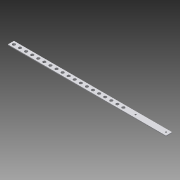
# Autodesk Inventor part: bottom clamper arm
Saved by Autodesk Inventor 2015 (Build 190159000, 159)
## iProperties
Created: 2015-03-29
Part Number: bottom clamper arm
Material: Aluminum 6061
Document SubType Name: Modeling
Designer: Jarod
Density: 2.7 g/cm^3
Appearance: Aluminum - Flat
Author: Jarod
Autodesk Inventor part; units mm, degrees
ref_plane "YZ Plane" through (0, 0, 0) normal (1, 0, 0) x (0, 1, 0)
ref_plane "XZ Plane" through (0, 0, 0) normal (0, 1, 0) x (-1, 0, 0)
ref_plane "XY Plane" through (0, 0, 0) normal (0, 0, 1) x (1, 0, 0)
sketch "Sketch1" plane through (0, 0, 0) normal (1, 0, 0) x (0, 1, 0)
  line L0 (0, 0) -> (-3.175, 0)
  line L1 (-3.175, 0) -> (-3.175, 25.4)
  line L2 (-3.175, 25.4) -> (0, 25.4)
  line L3 (0, 25.4) -> (0, 0)
  line L4 (0, 0) -> (-25.4, 0)
  line L5 (-25.4, 0) -> (-25.4, 3.175)
  line L6 (-25.4, 3.175) -> (0, 3.175)
  line L7 (0, 3.175) -> (0, 0)
  dimension "d0" = 3.175
  dimension "d1" = 25.4
  dimension "d2" = 25.4
  dimension "d3" = 3.175
  constraints: 16 end point, 4 parallel, 2 horizontal, 2 perpendicular
  measures "d0" distance of L1.end L2.end
  measures "d1" distance of L0.end L1.end
  measures "d2" distance of L5.end L6.end
  measures "d3" distance of L4.end L5.end
extrude "Extrusion1" add sketch "Sketch1" along normal blind 660.4
sketch "Sketch2" plane through (0, -25.4, 3.175) normal (0, 0, 1) x (1, 0, 0)
  line L0 (660.4, 22.225) -> (0, 22.225) projected
  line L1 (0, 22.225) -> (0, 0) projected
  line L2 (0, 0) -> (660.4, 0) projected
  line L3 (660.4, 22.225) -> (660.4, 0) projected
  line L4 (660.4, 0) -> (482.6, 0)
  line L5 (482.6, 0) -> (482.6, 22.225)
  line L6 (482.6, 22.225) -> (660.4, 22.225)
  line L7 (660.4, 22.225) -> (660.4, 0)
  point P0 (0, 25.4)
  dimension "d6" = 177.8
  dimension "d7" = 22.225
  constraints: 8 end point, 2 parallel, 1 horizontal, 1 perpendicular
  measures "d6" distance of L5.end L6.end
  measures "d7" distance of L4.end L5.end
extrude "Extrusion2" cut sketch "Sketch2" against normal blind 25.4 contours L3 L2 L5 L0
sketch "Sketch3" plane through (0, 0, 25.4) normal (0, 1, 0) x (1, 0, 0)
  line L0 (0, 25.4) -> (0, 0) projected
  line L1 (0, 0) -> (660.4, 0) projected
  line L2 (660.4, 25.4) -> (660.4, 0) projected
  line L3 (0, 25.4) -> (660.4, 25.4) projected
  point P0 (647.7, 12.7)
  point P1 (520.7, 12.7)
  dimension "d10" = 12.7
  dimension "d11" = 12.7
  dimension "d12" = 139.7
  dimension "d13" = 12.7
  measures "d10" distance from line of L3 point (647.7, 12.7)
  measures "d11" distance from line of L2 point (647.7, 12.7)
  measures "d12" distance from line of point (520.7, 12.7) L2
  measures "d13" distance from line of L3 point (520.7, 12.7)
hole "Hole1" at (647.7, 0, 12.7) at (520.7, 0, 12.7) direction (0, -1, 0) diameter 6.7469 end through all
sketch "Sketch4" plane through (0, -25.4, 0) normal (0, 0, -1) x (-1, 0, 0)
  line L0 (-660.4, 22.225) -> (-482.6, 22.225) projected
  line L1 (-482.6, 22.225) -> (-482.6, 0) projected
  line L2 (0, 0) -> (-482.6, 0) projected
  line L3 (0, 0) -> (0, 25.4) projected
  line L4 (0, 25.4) -> (-660.4, 25.4) projected
  line L5 (-660.4, 22.225) -> (-660.4, 25.4) projected
  line L6 (0, 0) -> (-482.6, 0)
  line L7 (-482.6, 0) -> (-482.6, 12.7)
  line L8 (-482.6, 12.7) -> (0, 12.7)
  line L9 (0, 12.7) -> (0, 0)
  dimension "d21" = 482.6
  dimension "d22" = 12.7
  constraints: 8 end point, 2 parallel, 1 horizontal, 1 perpendicular
  measures "d21" distance of L7.end L8.end
  measures "d22" distance of L6.end L7.end
extrude "Extrusion3" cut sketch "Sketch4" against normal blind 25.4 contours L8 L3 L2 L1
sketch "Sketch5" plane through (0, 0, 25.4) normal (0, 1, 0) x (1, 0, 0)
  circle A0 centre (647.7, 12.7) radius 3.3734 projected
  circle A1 centre (520.7, 12.7) radius 3.3734 projected
  line L0 (0, 25.4) -> (0, 0) projected
  line L1 (0, 0) -> (660.4, 0) projected
  line L2 (660.4, 25.4) -> (660.4, 0) projected
  line L3 (0, 25.4) -> (660.4, 25.4) projected
  point P0 (12.7, 12.7)
  dimension "d25" = 12.7
  dimension "d26" = 12.7
  measures "d25" distance from line of L3 point (12.7, 12.7)
  measures "d26" distance from line of L0 point (12.7, 12.7)
hole "Hole2" at (12.7, 0, 12.7) direction (0, -1, 0) diameter 12.7 end through all
pattern_linear "Rectangular Pattern1" count 19 spacing 25.4 along (1, 0, 0) of "Hole2"
body "Solid1"
